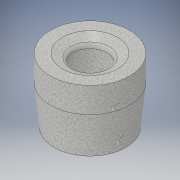
# Autodesk Inventor part: graphite
Saved by Autodesk Inventor 2017 (Build 210142000, 142)
## iProperties
Created: 2016-07-25
Part Number: graphite
Material: GFRC
Document SubType Name: Modeling
Designer: Jared
Density: 1.7 g/cm^3
Appearance: Flat - Polished Gray
Author: Jared
Autodesk Inventor part; units mm, degrees
ref_plane "YZ Plane" through (0, 0, 0) normal (1, 0, 0) x (0, 1, 0)
ref_plane "XZ Plane" through (0, 0, 0) normal (0, 1, 0) x (-1, 0, 0)
ref_plane "XY Plane" through (0, 0, 0) normal (0, 0, 1) x (1, 0, 0)
sketch "Sketch1" plane through (0, 0, 0) normal (0, 0, 1) x (1, 0, 0)
  line L0 (0, 25.4) -> (-28.702, 25.4) construction
  line L1 (0, 25.4) -> (-93.98, 25.4) construction
  line L2 (-93.98, 25.4) -> (-90.805, 25.4) construction
  line L3 (-90.805, 25.4) -> (-84.455, 22.4389) construction
  line L4 (-90.805, 25.4) -> (-90.805, 22.4389) construction
  line L5 (-90.805, 0) -> (-93.98, 0)
  line L6 (-28.702, 59.6457) -> (-28.702, -91.9304) construction
  arc A0 (-28.9184, -9.248) -> (-32.3684, -1.8494) centre (-35.052, -7.6045) ccw
  line L7 (-74.93, -180.9657) -> (-28.702, -8.4405)
  line L8 (-90.805, 25.4) -> (-90.805, 0)
  line L9 (-90.805, 25.4) -> (-32.3684, -1.8494)
  line L10 (-28.702, -7.6045) -> (-60.452, -7.6045) construction
  line L11 (-60.452, -126.9331) -> (-54.102, -126.9331) construction
  line L12 (-54.102, -126.9331) -> (-54.102, -103.2346) construction
  line L13 (-54.102, -103.2346) -> (-60.452, -103.2346)
  line L14 (-60.452, 11.2462) -> (-60.452, 1.7212) construction
  line L15 (-60.452, 11.2462) -> (-60.452, 4.7154) construction
  line L16 (-60.452, 4.7154) -> (-46.4468, 4.7154)
  line L17 (-93.98, 0) -> (-93.98, -12.7) construction
  line L18 (-60.452, -12.7) -> (-73.152, -12.7) construction
  line L19 (-93.98, -12.7) -> (-93.98, -25.4) construction
  line L20 (-93.98, -25.4) -> (-93.98, -88.9) construction
  line L21 (-93.98, -88.9) -> (-81.28, -88.9) construction
  line L22 (-81.28, -88.9) -> (-81.28, -25.4) construction
  line L23 (-93.98, -25.4) -> (-81.28, -25.4)
  line L24 (-81.28, -25.4) -> (-81.28, -88.9)
  line L25 (-81.28, -88.9) -> (-93.98, -88.9)
  line L26 (-93.98, -12.7) -> (-73.152, -12.7)
  line L27 (-73.152, -138.7824) -> (-63.627, -138.7824)
  line L28 (-81.28, -88.9) -> (-81.28, -180.9657)
  line L29 (-81.28, -180.9657) -> (-74.93, -180.9657)
  line L30 (-73.152, -12.7) -> (-73.152, -138.7824)
  line L31 (-87.63, -25.4) -> (-87.63, -31.3436)
  line L32 (-87.63, -31.3436) -> (-93.98, -31.3436)
  line L33 (-93.98, 0) -> (-93.98, -25.4)
  line L34 (-93.98, -31.3436) -> (-93.98, -88.9)
  line L35 (-87.63, -155.5657) -> (-87.63, -216.5135)
  line L36 (-28.9184, -9.248) -> (-84.455, -216.5135)
  line L37 (-84.455, -216.5135) -> (-87.63, -216.5135)
  line L38 (-81.28, -155.5657) -> (-87.63, -155.5657)
  line L39 (-66.802, -38.1) -> (-73.152, -38.1)
  line L40 (-66.802, -38.1) -> (-66.802, 4.7154)
  line L41 (-66.802, 4.7154) -> (-60.452, 4.7154)
  line L42 (-66.802, -38.1) -> (-60.452, -103.2346)
  line L43 (-60.452, 11.2462) -> (-60.452, 4.7154) construction
  line L44 (-60.452, -7.6045) -> (-60.452, -12.7) construction
  line L45 (-60.452, -103.2346) -> (-60.452, -126.9331) construction
  line L46 (0, -319.0244) -> (0, 122.7573) projected
  point P0 (0, 0)
  point P1 (-93.98, -255.9127)
  point P2 (-88.7095, 22.4389)
  dimension "d0" = 28.702
  dimension "d1" = 93.98
  dimension "d2" = 3.175
  dimension "d3" = 25
  dimension "d5" = 25.4
  dimension "d6" = 25.4
  dimension "d8" = 12.7
  dimension "d12" = 31.75
  dimension "d13" = 6.35
  dimension "d16" = 12.7
  dimension "d17" = 12.7
  dimension "d18" = 12.7
  dimension "d19" = 63.5
  dimension "d20" = 12.7
  dimension "d22" = 9.525
  dimension "d23" = 6.35
  dimension "d25" = 5.9436
  dimension "d27" = 3.175
  dimension "d28" = 6.35
  dimension "d29" = 25.4
  dimension "d30" = 107.95
  dimension "d31" = 6.35
  dimension "d32" = 25.4
  dimension "d33" = 20.3552
  dimension "d34" = 15
  constraints: 92 end point, 25 perpendicular, 18 point on line, 15 vertical, 5 tangent, 5 vertical alignment, 4 horizontal, 3 point on circle, 2 midpoint, 1 centre point, 1 collinear
  measures "d0" distance of L0.start L0.end
  measures "d1" distance of L0.start L1.end
  measures "d2" distance of L2.end L1.end
  measures "d3" angle of L1 L3
  measures "d5" distance of point (0, 0) L0.start
  measures "d6" distance of L2.end L5.start
  measures "d8" diameter of A0
  measures "d12" distance of L10.end L10.start
  measures "d13" distance of L11.start L11.end
  measures "d16" distance of L5.end L17.end
  measures "d17" distance of L18.start L18.end
  measures "d18" distance of L17.end L19.end
  measures "d19" distance of L20.end L19.end
  measures "d20" distance of L20.end L21.end
  measures "d22" distance of L27.start L27.end
  measures "d23" distance of L28.end L7.start
  measures "d25" distance of L31.start L31.end
  measures "d27" distance of L35.end L36.end
  measures "d28" distance of L38.start L35.start
  measures "d29" distance from line of L28.end L38
  measures "d30" distance of L13.end L15.end
  measures "d31" distance between parallel lines of L30 L40
  measures "d32" distance from line of L18.end L39
  measures "d33" distance of L16.end L40.end
  measures "d34" angle of L6 L36
revolve "Revolution1" add sketch "Sketch1" angle 360 about axis through (0, -10, 0) along (0, 1, 0) contours L9 A0 L7 L13 L42 L40 L41 L16
body "Solid1"
